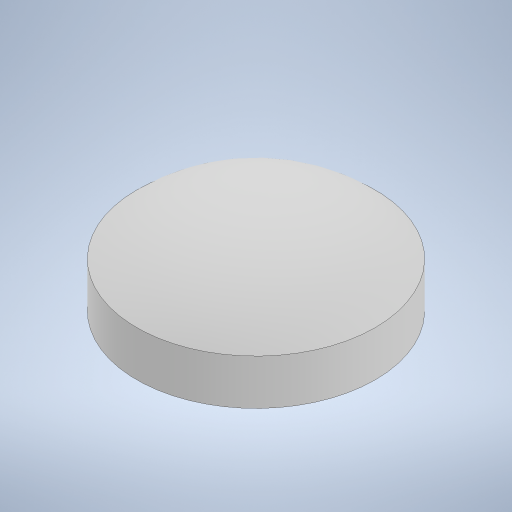
# Autodesk Inventor part: Деталь 4
Saved by Autodesk Inventor 2024.2 (Build 282272000, 272)
## iProperties
Created: 2024-10-18
Part Number: Деталь 4
Material: Типовые
Document SubType Name: Modeling
Designer: ASUS
Density: 1 g/cm^3
Appearance: По умолчанию
Author: ASUS
Autodesk Inventor part; units mm, degrees
ref_plane "YZ Plane" through (0, 0, 0) normal (1, 0, 0) x (0, 1, 0)
ref_plane "XZ Plane" through (0, 0, 0) normal (0, 1, 0) x (-1, 0, 0)
ref_plane "XY Plane" through (0, 0, 0) normal (0, 0, 1) x (1, 0, 0)
sketch "Эскиз1" plane through (0, 0, 0) normal (0, 0, 1) x (1, 0, 0)
  line L0 (0, 0) -> (20, 0)
  line L1 (0, 0) -> (0, 16)
  arc A0 (20, 7.5959) -> (0, 16) centre (0, -12) ccw
  line L2 (20, 0) -> (20, 7.5959)
  line L3 (0, 0) -> (-20, 0)
  arc A1 (0, 16) -> (-20, 7.5959) centre (0, -12) ccw
  line L4 (-20, 0) -> (-20, 7.5959)
  constraints: 10 end point, 4 point on circle, 2 centre point, 2 symmetric about line, 2 vertical, 1 horizontal, 1 other
revolve "Вращение1" add sketch "Эскиз1" angle 360 about axis through (0, 0, 0) along (0, 1, 0) contours L3 L4 A1 L1
